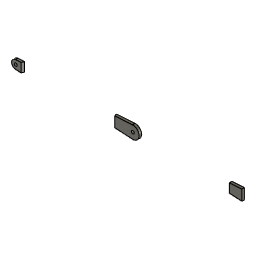
link2 v3 (Autodesk Fusion 360 design; units mm, degrees)
Autodesk Fusion 360 part; units mm, degrees
sketch "Sketch1" plane through (0, 0, 0) normal (0, 1, 0) x (1, 0, 0)
  line L0 (0, 0) -> (200, 0)
  line L1 (0, 0) -> (200.6428, -12.4652)
  line L2 (0, 0) -> (201.0296, 0) construction
  line L3 (0, 0) -> (199.7661, 12.4107)
  line L4 (0, 0) -> (200.1513, 0) construction
  circle A0 centre (32.2546, 0) radius 2
  line L5 (30.2546, 0) -> (35.2746, 0)
  line L6 (35.2746, -2.1915) -> (35.2746, 2.1915)
  circle A1 centre (32.2546, 0) radius 0.7
  dimension "d1" = 3.555
  dimension "d2" = 3.555
  dimension "d3" = 4
  dimension "d4" = 5.02
  dimension "d5" = 1.4
  constraint coincident L0.start L1.start
  constraint horizontal L0
  constraint horizontal L2
  constraint horizontal L4
  constraint coincident L4 A0.centre
  constraint tangent L1 A0
  constraint coincident A0 L5.start
  constraint coincident L0 L5.start
  constraint parallel L0 L5
  constraint coincident L1 L6.start
  constraint coincident L3 L6.end
  constraint coincident L5.end L6
  constraint perpendicular L2 L6
  constraint concentric A0 A1
  measures "d1" angle of L1 L2
  measures "d2" angle of L3 L4
  measures "d3" diameter of A0
  measures "d4" distance of L5.start L5.end
  measures "d5" diameter of A1
extrude "Extrude1" add sketch "Sketch1" along normal blind 1.2 contours L0 A0 L5 A1 | L0 A0 L5 A1 | L0 L1 A0 L5 L6 | L0 L3 A0 L5 L6 makes body 1
sketch "Sketch2" plane through (0, 0, 0) normal (0, -1, 0) x (1, 0, 0)
  circle A0 centre (32.2546, 0) radius 0.7
  arc A1 (32.1306, 1.9962) -> (32.1306, -1.9962) centre (32.2546, 0) ccw
  line L0 (32.1306, -1.9962) -> (35.2746, -2.1915)
  line L1 (35.2746, -2.1915) -> (35.2746, 2.1915)
  line L2 (35.2746, 2.1915) -> (32.1306, 1.9962)
  line L3 (30.2546, 0) -> (34.8146, 0)
  line L4 (34.8146, 0) -> (34.8146, 2.1629)
  line L5 (34.8146, 0) -> (34.8146, -2.1629)
  dimension "d8" = 4.56
  constraint midpoint A1 L3.start
  constraint horizontal L3
  constraint coincident L2 L4.end
  constraint perpendicular L3 L4
  constraint coincident L0 L5.end
  constraint perpendicular L3 L5
  measures "d8" distance of L3.start L3.end
sketch "Sketch3" plane through (0, 0, 0) normal (-0.062007, 0, 0.998076) x (0, -1, 0)
  line L0 (0, 32.1926) -> (0, 35.3426)
  line L1 (0, 35.3426) -> (-1.2, 35.3426)
  line L2 (-1.2, 35.3426) -> (-1.2, 32.1926)
  line L3 (-1.2, 32.1926) -> (0, 32.1926)
  line L4 (-1.2, 35.3426) -> (0, 34.88)
  constraint coincident L1.end L2.start
  constraint coincident L0 L4.end
sweep "Sweep1" cut profiles "Sketch2" path "Sketch3" along L4 section 1 contours L0 L1 L2 L4 L5 bodies 1
extrude "Extrude2" add 1 faces at (35.1213, 0.3985, -2.1629) along direction (0.061936, -0.047662, 0.996941) blind 0.05 on bodies 1 bodies 1
sweep "Sweep2" cut 1 faces at (35.1244, 0.3961, -2.1131) along 1 edges at (34.8162, -0.0012, -2.138) on bodies 1 bodies 1
sweep "Sweep3" cut 1 faces at (35.2746, 0.7985, -2.1724) along 1 edges at (35.0446, 0.5978, -2.1486) on bodies 1 bodies 1
sketch "Sketch4" plane through (0, 0, 0) normal (0, -1, 0) x (1, 0, 0)
  line L0 (34.8146, -2.1629) -> (34.8146, 2.1629)
  line L1 (34.8146, 2.1629) -> (32.1306, 1.9962)
  arc A0 (32.1306, 1.9962) -> (32.1306, -1.9962) centre (32.2546, 0) ccw
  line L2 (32.1306, -1.9962) -> (34.8146, -2.1629)
  circle A1 centre (32.2546, 0) radius 0.7
  line L3 (40, 0) -> (140, 0)
  line L4 (40, 0) -> (139.8081, 6.192)
  line L5 (40, 0) -> (140, 0) construction
  line L6 (40, 0) -> (139.8081, -6.192)
  line L7 (40, 0) -> (140, 0) construction
  circle A2 centre (88.45, 0) radius 3
  line L8 (91.45, 0) -> (79.34, 0)
  line L9 (79.34, 2.4406) -> (79.34, -2.4406)
  circle A3 centre (88.45, 0) radius 0.7
  dimension "d29" = 100
  dimension "d30" = 3.55
  dimension "d31" = 100
  dimension "d32" = 3.55
  dimension "d33" = 100
  dimension "d34" = 6
  dimension "d35" = 12.11
  dimension "d36" = 1.4
  constraint horizontal L3
  constraint horizontal L5
  constraint horizontal L7
  constraint coincident L3 A2.centre
  constraint tangent L4 A2
  constraint coincident L7 L8.start
  constraint coincident A2 L8.start
  constraint parallel L5 L8
  constraint coincident L4 L9.start
  constraint coincident L6 L9.end
  constraint coincident L8.end L9
  constraint perpendicular L8 L9
  constraint concentric A2 A3
  measures "d29" distance of L3.start L3.end
  measures "d30" angle of L4 L5
  measures "d31" distance of L3.start L4.end
  measures "d32" angle of L6 L7
  measures "d33" distance of L3.start L6.end
  measures "d34" diameter of A2
  measures "d35" distance of L8.start L8.end
  measures "d36" diameter of A3
extrude "Extrude3" add sketch "Sketch4" against normal blind 1.2 separate body contours L3 L4 A2 L8 L9 | L3 L6 A2 L8 L9 | L3 A2 L8 A3 | L3 A2 L8 A3 makes body 2
sketch "Sketch5" plane through (0, 0, 0) normal (0, -1, 0) x (1, 0, 0)
  circle A0 centre (88.45, 0) radius 0.7
  line L0 (79.34, 2.4406) -> (79.34, -2.4406)
  line L1 (79.34, -2.4406) -> (88.2642, -2.9942)
  arc A1 (88.2642, -2.9942) -> (88.2642, 2.9942) centre (88.45, 0) ccw
  line L2 (88.2642, 2.9942) -> (79.34, 2.4406)
  line L3 (88.45, 0) -> (79.79, 0)
  line L4 (79.79, 2.4685) -> (79.79, -2.4685)
  dimension "d39" = 8.66
  constraint coincident A0.centre A1.centre
  constraint horizontal L3
  constraint coincident L2 L4.start
  constraint coincident L1 L4.end
  constraint perpendicular L3 L4
  constraint coincident L3.end L4
  measures "d39" distance of A0.centre L3.end
sketch "Sketch6" plane through (0.1534, 0, 2.472) normal (-0.06192, 0, -0.998081) x (0, -1, 0)
  line L0 (0, -88.2802) -> (0, -79.3388)
  line L1 (0, -79.3388) -> (-1.2, -79.3388)
  line L2 (-1.2, -79.3388) -> (-1.2, -88.2802)
  line L3 (-1.2, -88.2802) -> (0, -88.2802)
  line L4 (-1.2, -79.3388) -> (0, -79.7897)
  point P0 (0, -79.7897)
  constraint coincident L1.end L2.start
  constraint coincident L0 P0
  constraint coincident P0 L4.end
sweep "Sweep4" cut profiles "Sketch6" path "Sketch5" along L4 section 1 contours L0 L1 L4 bodies 2
sketch "Sketch7" plane through (0, 0, 0) normal (0, 1, 0) x (1, 0, 0)
  line L0 (100, 0) -> (149.9038, -3.1003)
  line L1 (100, 0) -> (150, 0) construction
  line L2 (100, 0) -> (149.9038, 3.1003)
  line L3 (100, 0) -> (150, 0) construction
  circle A0 centre (132.2546, 0) radius 2
  line L4 (130.2546, 0) -> (134.8146, 0)
  line L5 (134.8146, -2.1629) -> (134.8146, 2.1629)
  line L6 (134.8146, -2.1629) -> (140.7931, -2.5343)
  line L7 (140.7931, -2.5343) -> (140.7931, 2.5343)
  dimension "d46" = 50
  dimension "d47" = 3.555
  dimension "d48" = 3.555
  dimension "d49" = 50
  dimension "d50" = 4
  dimension "d51" = 4.56
  dimension "d52" = 5.99
  constraint horizontal L1
  constraint horizontal L3
  constraint coincident L1 A0.centre
  constraint tangent L0 A0
  constraint coincident A0 L4.start
  constraint coincident L3 L4.start
  constraint parallel L3 L4
  constraint coincident L0 L5.start
  constraint coincident L2 L5.end
  constraint coincident L4.end L5
  constraint perpendicular L1 L5
  constraint parallel L0 L6
  constraint coincident L2 L7.end
  constraint perpendicular L1 L7
  measures "d46" distance of L0.start L0.end
  measures "d47" angle of L0 L1
  measures "d48" angle of L2 L3
  measures "d49" distance of L0.start L2.end
  measures "d50" diameter of A0
  measures "d51" distance of L4.start L4.end
  measures "d52" distance of L5.start L6.end
extrude "Extrude1'" add sketch "Sketch7" along normal blind 1.2 separate body contours L0 L2 L5 L6 L7 makes body 3 in component "Component"
component "Component" placed x (1, 0, 0) y (0, 1, 0) z (0, 0, 1) at (0, 0, 0)
